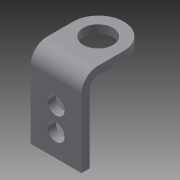
# Autodesk Inventor part: RSL plate
Saved by Autodesk Inventor 2015 (Build 190159000, 159)
## iProperties
Created: 2015-01-25
Part Number: RSL plate
Material: Generic
Document SubType Name: Sheet Metal
Designer: chapale16
Density: 1 g/cm^3
Sheet Metal Rule: Default
Appearance: Default
Author: chapale16
Autodesk Inventor part; units mm, degrees
ref_plane "YZ Plane" through (0, 0, 0) normal (1, 0, 0) x (0, 1, 0)
ref_plane "XZ Plane" through (0, 0, 0) normal (0, 1, 0) x (-1, 0, 0)
ref_plane "XY Plane" through (0, 0, 0) normal (0, 0, 1) x (1, 0, 0)
sketch "Sketch1" plane through (0, 0, 0) normal (0, 1, 0) x (-1, 0, 0)
  line L0 (0, 0) -> (19.05, 0)
  line L1 (19.05, 0) -> (19.05, -25.4)
  line L2 (19.05, -25.4) -> (0, -25.4)
  line L3 (0, -25.4) -> (0, 0)
  dimension "d0" = 25.4
  dimension "d1" = 19.05
  measures "d0" distance of L2.end L0.start
  measures "d1" distance of L1.end L2.end
extrude "Plate1" add sketch "Sketch1" along normal blind 3.048
sketch "Sketch2" plane through (-19.05, 3.048, -3.048) normal (0, 0, 1) x (1, 0, 0)
  line L0 (19.05, 0) -> (0, 0)
  line L1 (0, 0) -> (0, -31.75)
  line L2 (0, -31.75) -> (19.05, -31.75)
  line L3 (19.05, -31.75) -> (19.05, 0)
  constraints: 6 end point, 1 horizontal, 1 perpendicular, 1 vertical
edge flange "Flange1" height 31.75 angle 90 thickness 3.048 bend radius 3.048 thickness toward (0, 0, 1) relief tear relief width 3.048 relief depth 1.524 edges at (-9.525, 0, 0) wall of the first edge with corners at (0, 3.048, -3.048) (-19.05, 3.048, -3.048) (-19.05, -28.702, -3.048) (0, -28.702, -3.048)
bend "Bend1"
corner "Corner1"
sketch "Sketch3" plane through (0, 3.048, 0) normal (0, 1, 0) x (1, 0, 0)
  line L0 (-19.05, 6.096) -> (-19.05, 25.4) projected
  line L1 (-19.05, 25.4) -> (0, 25.4) projected
  circle A0 centre (-9.525, 15.748) radius 5.5563
  point P0 (0, 0)
  dimension "d13" = 11.1125
  constraints: 1 centre point
  measures "d13" diameter of A0
extrude "Cut1" cut sketch "Sketch3" against normal blind 3.048
fillet "Corner Round1" radius 9.525 2 edges at (0, 1.524, -25.4) (-19.05, 1.524, -25.4)
sketch "Sketch5" plane through (-19.05, -28.702, 0) normal (0, 0, 1) x (1, 0, 0)
  line L0 (0, 0) -> (0, 25.654) projected
  line L1 (19.05, 0) -> (0, 0) projected
  line L2 (19.05, 25.654) -> (19.05, 0) projected
  line L3 (19.05, 25.654) -> (0, 25.654) projected
  line L4 (0, 25.654) -> (19.05, 25.654) projected
  line L5 (9.525, 25.654) -> (9.525, 17.1027)
  line L6 (9.525, 17.1027) -> (9.525, 8.5429)
  circle A0 centre (9.525, 17.1027) radius 3.175
  circle A1 centre (9.525, 8.5429) radius 3.175
  point P0 (19.05, 28.702)
  dimension "d17" = 8.5513
  dimension "d18" = 8.5598
  dimension "d19" = 6.35
  dimension "d20" = 6.35
  constraints: 4 end point, 2 centre point, 2 coincident, 1 midpoint, 1 point on line, 1 vertical
  measures "d17" distance of L5.start L5.end
  measures "d18" distance of L5.end L6.end
  measures "d19" diameter of A0
  measures "d20" diameter of A1
extrude "Cut2" cut sketch "Sketch5" against normal blind 3.048 contours A0 L6 L5 | L5 L6 A0 | A1
equation "\"d14\" = Thickness"
equation "\"d21\" = Thickness"
equation "\"d3\" = BendReliefWidth"
equation "\"d4\" = BendReliefDepth"
equation "\"d5\" = MinimumRemnant"
equation "\"d6\" = BendRadius"
equation "\"d9\" = BendRadius"
equation "\"d10\" = CornerReliefSize"
equation "\"d11\" = GapSize"
equation "\"d12\" = JacobiRadiusSize"
equation "\"BendRadius\" = Thickness"
equation "\"BendReliefWidth\" = Thickness"
equation "\"BendReliefDepth\" = 0.5 * Thickness"
equation "\"CornerReliefSize\" = 4 * Thickness"
equation "\"MinimumRemnant\" = 2 * Thickness"
equation "\"TransitionRadius\" = BendRadius"
equation "\"JacobiRadiusSize\" = BendRadius"
equation "\"GapSize\" = Thickness"
equation "\"d2\" = BendRadius"
equation "\"Thickness\" = 3.048"
body "Solid1"
